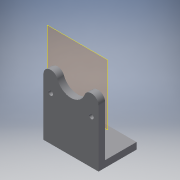
# Autodesk Inventor part: Shelf Braket
Saved by Autodesk Inventor 2019.4 (Build 234330000, 330)
## iProperties
Created: 2021-04-16
Part Number: Shelf Braket
Material: Generic
Document SubType Name: Modeling
Designer: Ian
Density: 1 g/cm^3
Appearance: Default
Author: Ian
Autodesk Inventor part; units mm, degrees
ref_plane "YZ Plane" through (0, 0, 0) normal (1, 0, 0) x (0, 1, 0)
ref_plane "XZ Plane" through (0, 0, 0) normal (0, 1, 0) x (-1, 0, 0)
ref_plane "XY Plane" through (0, 0, 0) normal (0, 0, 1) x (1, 0, 0)
ref_plane "Work Plane1" through (0, 0, 0) normal (0, 0, 1) x (1, 0, 0)
sketch "Sketch1" plane through (0, 0, 0) normal (0, 0, 1) x (1, 0, 0)
  circle A0 centre (0, 0) radius 11 projected
  circle A1 centre (-15.5, -15.5) radius 1.75 projected
  circle A2 centre (15.5, -15.5) radius 1.75 projected
  circle A3 centre (15.5, 15.5) radius 1.75 projected
  circle A4 centre (-15.5, 15.5) radius 1.75 projected
  line L0 (-21, 21) -> (21, 21) projected
  line L1 (-21, -21) -> (-21, 21) projected
  line L2 (21, -21) -> (-21, -21) projected
  line L3 (21, 21) -> (21, -21) projected
  line L4 (40.7911, -42.1) -> (-34.1821, -42.1) projected
  line L5 (21, -44.1) -> (-21, -44.1)
  arc A5 (-10.3333, -3.7712) -> (-21, -5.6569) centre (-15.5, -5.6569) ccw
  arc A6 (-10.3333, -3.7712) -> (10.3333, -3.7712) centre (0, 0) ccw
  arc A7 (21, -5.6569) -> (10.3333, -3.7712) centre (15.5, -5.6569) ccw
  line L6 (-21, -5.6569) -> (-21, -44.1)
  line L7 (21, -5.6569) -> (21, -44.1)
  line L8 (-21, -21) -> (21, -21)
  line L9 (21, -21) -> (21, -49.1)
  line L10 (21, -49.1) -> (-21, -49.1)
  line L11 (-21, -49.1) -> (-21, -21)
  point P0 (0, 0)
  dimension "d0" = 2
  dimension "d1" = 5
  constraints: 14 end point, 8 point on circle, 4 point on line, 4 tangent, 3 centre point, 3 parallel, 2 vertical alignment, 1 collinear, 1 concentric, 1 horizontal, 1 perpendicular
  measures "d0" distance between parallel lines of L4 L5
  measures "d1" distance between parallel lines of L5 L10
extrude "Extrusion1" add sketch "Sketch1" along normal blind 5 contours A0 A7 L3 L2 L1 A5 | L2 L7 L4 L6 | L4 L7 L5 L6 | L5 L9 L10 L11
sketch "Sketch2" plane through (0, 0, 0) normal (0, 0, -1) x (-1, 0, 0)
  line L0 (-21, -49.1) -> (21, -49.1) projected
  line L1 (21, -5.6569) -> (21, -49.1) projected
  line L2 (-21, -49.1) -> (21, -49.1)
  line L3 (21, -49.1) -> (21, -44.1)
  line L4 (21, -44.1) -> (-21, -44.1)
  line L5 (-21, -44.1) -> (-21, -49.1)
  point P0 (0, 0)
  dimension "d4" = 5
  constraints: 8 end point, 2 parallel, 1 horizontal, 1 perpendicular, 1 point on line
  measures "d4" distance between parallel lines of L0 L4
extrude "Extrusion2" add sketch "Sketch2" along normal blind 24
body "Solid1"
